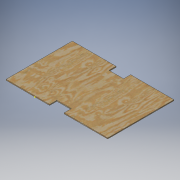
# Autodesk Inventor part: skid plate
Saved by Autodesk Inventor 2016 (Build 200138000, 138)
## iProperties
Created: 2016-02-03
Part Number: skid plate
Material: Generic
Document SubType Name: Modeling
Designer: Andrew
Density: 1 g/cm^3
Appearance: Plywood - Weathered
Author: Andrew
Autodesk Inventor part; units mm, degrees
ref_plane "YZ Plane" through (0, 0, 0) normal (1, 0, 0) x (0, 1, 0)
ref_plane "XZ Plane" through (0, 0, 0) normal (0, 1, 0) x (-1, 0, 0)
ref_plane "XY Plane" through (0, 0, 0) normal (0, 0, 1) x (1, 0, 0)
sketch "Sketch1" plane through (0, 0, 0) normal (0, 1, 0) x (-1, 0, 0)
  point P0 (0, 0)
sketch "Sketch2" plane through (0, 0, 0) normal (0, 1, 0) x (-1, 0, 0)
  line L0 (202.6839, 344.3242) -> (-508.5161, 344.3242)
  line L1 (-508.5161, 344.3242) -> (-508.5161, -119.2258)
  line L2 (-508.5161, -119.2258) -> (202.6839, -119.2258)
  line L3 (202.6839, -119.2258) -> (202.6839, 344.3242)
  point P0 (0, 0)
  dimension "d0" = 463.55
  dimension "d1" = 711.2
  constraints: 8 end point, 2 parallel, 1 horizontal, 1 perpendicular
  measures "d0" distance of L2.end L0.start
  measures "d1" distance of L1.end L2.end
extrude "Extrusion1" add sketch "Sketch2" along normal blind 6.35
sketch "Sketch3" plane through (0, 6.35, 0) normal (0, 1, 0) x (1, 0, 0)
  line L0 (102.1161, -344.3242) -> (203.7161, -344.3242)
  line L1 (203.7161, -344.3242) -> (203.7161, -293.5242)
  line L2 (203.7161, -293.5242) -> (102.1161, -293.5242)
  line L3 (102.1161, -293.5242) -> (102.1161, -344.3242)
  line L4 (-202.6839, 119.2258) -> (-202.6839, -344.3242) projected
  line L5 (508.5161, 119.2258) -> (-202.6839, 119.2258) projected
  line L6 (103.7036, 70.0133) -> (205.3036, 70.0133)
  line L7 (205.3036, 70.0133) -> (205.3036, 120.8133)
  line L8 (205.3036, 120.8133) -> (103.7036, 120.8133)
  line L9 (103.7036, 120.8133) -> (103.7036, 70.0133)
  line L10 (-202.6839, -344.3242) -> (508.5161, -344.3242) projected
  point P0 (0, 0)
  dimension "d4" = 50.8
  dimension "d5" = 101.6
  dimension "d6" = 304.8
  dimension "d8" = 50.8
  dimension "d9" = 101.6
  dimension "d10" = 0
  constraints: 16 end point, 4 parallel, 2 horizontal, 2 perpendicular
  measures "d4" distance of L2.end L0.start
  measures "d5" distance of L1.end L2.end
  measures "d6" distance between parallel lines of L4 L3
  measures "d8" distance of L8.end L6.start
  measures "d9" distance of L7.end L8.end
  measures "d10" distance between parallel lines of L0 L10
extrude "Extrusion2" cut sketch "Sketch3" against normal blind 6.35
sketch "Sketch4" plane through (-202.6839, 0, 344.3242) normal (0, 0, 1) x (1, 0, 0)
  point P0 (202.6839, 0)
body "Solid1"
